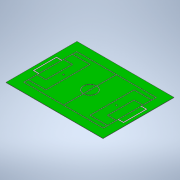
# Autodesk Inventor part: SoccerField_KidSize
Saved by Autodesk Inventor 2022 (Build 260153000, 153)
## iProperties
Created: 2022-10-30
Part Number: SoccerField_KidSize
Material: 一般
Document SubType Name: Modeling
Designer: Masato Kubotera
Density: 1 g/cm^3
Appearance: 既定
Author: Masato Kubotera
Autodesk Inventor part; units mm, degrees
ref_plane "YZ Plane" through (0, 0, 0) normal (1, 0, 0) x (0, 1, 0)
ref_plane "XZ Plane" through (0, 0, 0) normal (0, 1, 0) x (-1, 0, 0)
ref_plane "XY Plane" through (0, 0, 0) normal (0, 0, 1) x (1, 0, 0)
sketch "スケッチ1" plane through (0, 0, 0) normal (0, 0, 1) x (1, 0, 0)
  line L0 (-550, -402.5) -> (550, -402.5)
  line L1 (550, -402.5) -> (550, 402.5)
  line L2 (550, 402.5) -> (-550, 402.5)
  line L3 (-550, 402.5) -> (-550, -402.5)
  line L4 (-550, -402.5) -> (550, 402.5) construction
  line L5 (550, -402.5) -> (-550, 402.5) construction
  line L6 (550, 0) -> (-550, 0) construction
  line L7 (0, 402.5) -> (0, -402.5)
  line L8 (-447.5, -297.5) -> (447.5, -297.5)
  line L9 (447.5, -297.5) -> (447.5, -252.5)
  line L10 (447.5, 297.5) -> (-447.5, 297.5)
  line L11 (-447.5, 297.5) -> (-447.5, -297.5)
  line L12 (-447.5, -297.5) -> (447.5, 297.5) construction
  line L13 (447.5, -297.5) -> (-447.5, 297.5) construction
  line L14 (-452.5, -302.5) -> (452.5, -302.5)
  line L15 (452.5, -302.5) -> (452.5, -135)
  line L16 (452.5, 302.5) -> (-452.5, 302.5)
  line L17 (-452.5, 302.5) -> (-452.5, -302.5)
  line L18 (-452.5, -302.5) -> (452.5, 302.5) construction
  line L19 (452.5, -302.5) -> (-452.5, 302.5) construction
  line L20 (-450, -300) -> (450, -300) construction
  line L21 (450, -300) -> (450, 300) construction
  line L22 (450, 300) -> (-450, 300) construction
  line L23 (-450, 300) -> (-450, -300) construction
  line L24 (-450, -300) -> (450, 300) construction
  line L25 (450, -300) -> (-450, 300) construction
  line L26 (450, 130) -> (510, 130) construction
  line L27 (510, 130) -> (510, -130) construction
  line L28 (452.5, 125) -> (505, 125)
  line L29 (505, 125) -> (505, -125)
  line L30 (452.5, 135) -> (505, 135)
  line L31 (515, 135) -> (515, -135)
  line L32 (450, -130) -> (510, -130) construction
  line L33 (452.5, -125) -> (505, -125)
  line L34 (452.5, -135) -> (515, -135)
  line L35 (450, 150) -> (350, 150) construction
  line L36 (350, 150) -> (350, -150) construction
  line L37 (350, -150) -> (450, -150) construction
  line L38 (447.5, 152.5) -> (347.5, 152.5)
  line L39 (347.5, 152.5) -> (347.5, -152.5)
  line L40 (347.5, -152.5) -> (447.5, -152.5)
  line L41 (447.5, -147.5) -> (352.5, -147.5)
  line L42 (352.5, -147.5) -> (352.5, 147.5)
  line L43 (352.5, 147.5) -> (447.5, 147.5)
  line L44 (450, 250) -> (250, 250) construction
  line L45 (250, 250) -> (250, -250) construction
  line L46 (447.5, 252.5) -> (247.5, 252.5)
  line L47 (247.5, 252.5) -> (247.5, -252.5)
  line L48 (447.5, 247.5) -> (252.5, 247.5)
  line L49 (252.5, 247.5) -> (252.5, -247.5)
  line L50 (447.5, -252.5) -> (247.5, -252.5)
  line L51 (447.5, -247.5) -> (252.5, -247.5)
  line L52 (450, -250) -> (250, -250) construction
  arc A0 (2.5, 72.4569) -> (-2.5, 72.4569) centre (0, 0) ccw construction
  arc A1 (2.5, 77.4597) -> (-2.5, 77.4597) centre (0, 0) ccw construction
  circle A2 centre (0, 0) radius 75 construction
  line L53 (2.5, 297.5) -> (2.5, 77.4597)
  line L54 (-2.5, 297.5) -> (-2.5, 77.4597)
  line L55 (-7.5, 2.5) -> (-2.5, 2.5)
  line L56 (7.5, 2.5) -> (7.5, -2.5)
  line L57 (7.5, -2.5) -> (2.5, -2.5)
  line L58 (-7.5, -2.5) -> (-7.5, 2.5)
  line L59 (-7.5, 2.5) -> (7.5, -2.5) construction
  line L60 (7.5, 2.5) -> (-7.5, -2.5) construction
  line L61 (292.5, 2.5) -> (297.5, 2.5)
  line L62 (307.5, 2.5) -> (307.5, -2.5)
  line L63 (307.5, -2.5) -> (302.5, -2.5)
  line L64 (292.5, -2.5) -> (292.5, 2.5)
  line L65 (292.5, 2.5) -> (307.5, -2.5) construction
  line L66 (307.5, 2.5) -> (292.5, -2.5) construction
  line L67 (297.5, 7.5) -> (302.5, 7.5)
  line L68 (302.5, 7.5) -> (302.5, 2.5)
  line L69 (302.5, -7.5) -> (297.5, -7.5)
  line L70 (297.5, -7.5) -> (297.5, -2.5)
  line L71 (297.5, 7.5) -> (302.5, -7.5) construction
  line L72 (302.5, 7.5) -> (297.5, -7.5) construction
  line L73 (447.5, 247.5) -> (447.5, 252.5) construction
  line L74 (447.5, 252.5) -> (447.5, 297.5)
  line L75 (447.5, 147.5) -> (447.5, 152.5) construction
  line L76 (447.5, 152.5) -> (447.5, 247.5)
  line L77 (452.5, 125) -> (452.5, 135) construction
  line L78 (505, 135) -> (515, 135)
  line L79 (452.5, 135) -> (452.5, 302.5)
  line L80 (452.5, -125) -> (452.5, 125)
  line L81 (452.5, -135) -> (452.5, -125) construction
  line L82 (447.5, -152.5) -> (447.5, -147.5) construction
  line L83 (447.5, -147.5) -> (447.5, 147.5)
  line L84 (447.5, -252.5) -> (447.5, -247.5) construction
  line L85 (447.5, -247.5) -> (447.5, -152.5)
  line L86 (297.5, -2.5) -> (297.5, 2.5) construction
  line L87 (297.5, 2.5) -> (302.5, 2.5) construction
  line L88 (302.5, 2.5) -> (302.5, -2.5) construction
  line L89 (302.5, -2.5) -> (302.5, -7.5)
  line L90 (302.5, 2.5) -> (307.5, 2.5)
  line L91 (297.5, -2.5) -> (292.5, -2.5)
  line L92 (297.5, 2.5) -> (297.5, 7.5)
  line L93 (302.5, -2.5) -> (297.5, -2.5) construction
  arc A3 (58.5066, 42.8162) -> (2.5, 72.4569) centre (0, 0) ccw
  arc A4 (62.5415, 45.769) -> (2.5, 77.4597) centre (0, 0) ccw
  line L94 (2.5, 72.4569) -> (2.5, 2.5)
  line L95 (2.5, 77.4597) -> (2.5, 72.4569) construction
  line L96 (-2.5, 72.4569) -> (-2.5, 2.5)
  arc A5 (-2.5, 77.4597) -> (-2.5, -77.4597) centre (0, 0) ccw
  line L97 (-2.5, 77.4597) -> (-2.5, 72.4569) construction
  line L98 (-2.5, 2.5) -> (-2.5, -2.5) construction
  arc A6 (-2.5, 72.4569) -> (-2.5, -72.4569) centre (0, 0) ccw
  line L99 (2.5, -72.4569) -> (2.5, -77.4597) construction
  arc A7 (-2.5, -72.4569) -> (2.5, -72.4569) centre (0, 0) ccw construction
  arc A8 (-2.5, -77.4597) -> (2.5, -77.4597) centre (0, 0) ccw construction
  arc A9 (2.5, -77.4597) -> (62.5415, 45.769) centre (0, 0) ccw
  line L100 (2.5, -77.4597) -> (2.5, -297.5)
  line L101 (-2.5, -77.4597) -> (-2.5, -297.5)
  line L102 (-2.5, -72.4569) -> (-2.5, -77.4597) construction
  arc A10 (2.5, -72.4569) -> (58.5066, 42.8162) centre (0, 0) ccw
  line L103 (-2.5, 2.5) -> (0, 2.5) construction
  line L104 (0, 2.5) -> (2.5, 2.5) construction
  line L105 (2.5, 2.5) -> (2.5, -2.5) construction
  line L106 (2.5, 2.5) -> (7.5, 2.5)
  line L107 (2.5, -2.5) -> (-2.5, -2.5) construction
  line L108 (2.5, -2.5) -> (2.5, -72.4569)
  line L109 (-2.5, -2.5) -> (-2.5, -72.4569)
  line L110 (-2.5, -2.5) -> (-7.5, -2.5)
  point P0 (300, 0)
  point P1 (452.5, -127.5)
  point P2 (297.5, -2.5)
  point P3 (2.5, -2.5)
  point P4 (2.5, -72.4569)
  point P5 (2.5, 2.5)
  point P6 (-2.5, 2.5)
  point P7 (-2.5, 72.4569)
  point P8 (-2.5, -72.4569)
  point P9 (-2.5, -2.5)
  point P10 (-2.5, 77.4597)
  point P11 (452.5, -132.5)
  point P12 (0, 302.5)
  point P13 (0, -302.5)
  dimension "d1" = 100
  dimension "d2" = 5
  dimension "d3" = 5
  dimension "d4" = 100
  dimension "d5" = 600
  dimension "d6" = 900
  dimension "d7" = 260
  dimension "d8" = 10
  dimension "d9" = 10
  dimension "d10" = 60
  dimension "d11" = 5
  dimension "d12" = 5
  dimension "d13" = 300
  dimension "d14" = 100
  dimension "d15" = 5
  dimension "d16" = 5
  dimension "d17" = 200
  dimension "d18" = 500
  dimension "d19" = 150
  dimension "d20" = 5
  dimension "d21" = 145
  dimension "d22" = 5
  dimension "d23" = 5
  dimension "d24" = 15
  dimension "d25" = 5
  dimension "d26" = 5
  dimension "d27" = 15
  dimension "d28" = 15
  dimension "d29" = 150
  constraints: 222 end point, 84 perpendicular, 56 parallel, 21 point on circle, 18 midpoint, 17 point on line, 16 horizontal, 12 symmetric about line, 11 centre point, 3 coincident, 12 other
  measures "d1" distance between parallel lines of L1 L21
  measures "d2" distance between parallel lines of L9 L15
  measures "d3" distance between parallel lines of L16 L10
  measures "d4" distance between parallel lines of L2 L16
  measures "d5" distance of L20.end L21.end
  measures "d6" distance of L21.end L22.end
  measures "d7" distance between parallel lines of L32 L26
  measures "d8" distance between parallel lines of L29 L31
  measures "d9" distance between parallel lines of L30 L28
  measures "d10" distance between parallel lines of L21 L27
  measures "d11" distance between parallel lines of L38 L43
  measures "d12" distance between parallel lines of L39 L42
  measures "d13" distance between parallel lines of L37 L35
  measures "d14" distance between parallel lines of L21 L36
  measures "d15" distance between parallel lines of L48 L46
  measures "d16" distance between parallel lines of L47 L49
  measures "d17" distance between parallel lines of L45 L21
  measures "d18" distance of L44.end L45.end
  measures "d19" diameter of A2
  measures "d20" radial gap between concentric circles of A1 A0
  measures "d21" diameter of A0
  measures "d22" distance between parallel lines of L54 L53
  measures "d23" distance of L56.start L56.end
  measures "d24" distance of L56.end L58.start
  measures "d25" distance of L62.start L62.end
  measures "d26" distance of L69.start L69.end
  measures "d27" distance of L62.end L64.start
  measures "d28" distance of L69.end L67.start
  measures "d29" distance from line of L21 point (300, 0)
extrude "押し出し1" add sketch "スケッチ1" along normal blind 3 contours L7 L14 L15 L34 L31 L78 L30 L79 L16 L2 L1 L0 | L100 A9 A4 L53 L10 L74 L46 L47 L50 L9 L8 | L28 L29 L33 L80 | L38 L39 L40 L85 L51 L49 L48 L76 | L41 L42 L43 L83 | L106 L94 A3 A10 L108 L57 L56
extrude "押し出し2" add sketch "スケッチ1" along normal blind 3 separate body contours L7 L8 L9 L50 L47 L46 L74 L10 L16 L79 L30 L78 L31 L34 L15 L14 | L7 L10 L53 A4 A9 L100 L8 | L61 L92 L67 L68 L90 L62 L63 L89 L69 L70 L91 L64
mirror "ミラー1" about plane through (0, 0, 0) normal (1, 0, 0) bodies 2 1
equation "\"d3\" = d2"
equation "\"d4\" = d1"
equation "\"d11\" = d2"
equation "\"d12\" = d2"
equation "\"d15\" = d2"
equation "\"d16\" = d2"
equation "\"d20\" = d2"
equation "\"d21\" = d19 - d20"
equation "\"d22\" = d2"
equation "\"d23\" = d2"
equation "\"d24\" = 3 * d23"
equation "\"d25\" = d2"
equation "\"d26\" = d2"
equation "\"d27\" = d24"
equation "\"d28\" = d24"
